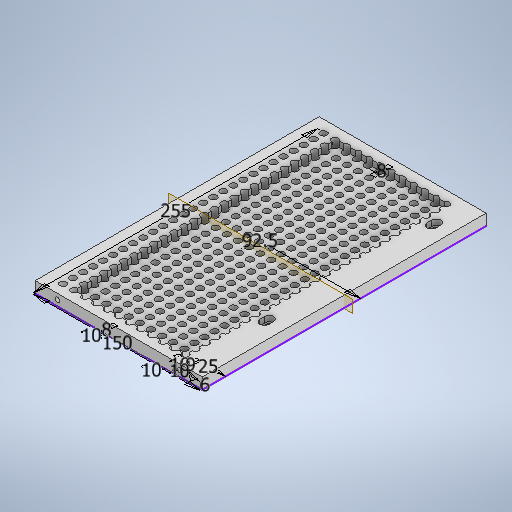
# Autodesk Inventor part: bottomplate
Saved by Autodesk Inventor 2025.2 (Build 292293000, 293)
## iProperties
Created: 2025-03-19
Part Number: bottomplate
Material: Generic
Document SubType Name: Modeling
Designer: m_kni
Density: 1 g/cm^3
Appearance: Default
Author: m_kni
Autodesk Inventor part; units mm, degrees
ref_plane "YZ Plane" through (0, 0, 0) normal (1, 0, 0) x (0, 1, 0)
ref_plane "XZ Plane" through (0, 0, 0) normal (0, 1, 0) x (-1, 0, 0)
ref_plane "XY Plane" through (0, 0, 0) normal (0, 0, 1) x (1, 0, 0)
sketch "Sketch1" plane through (0, 0, 0) normal (0, 1, 0) x (-1, 0, 0)
  line L0 (-74.8419, -127.4209) -> (75.1581, -127.4209)
  line L1 (75.1581, -127.4209) -> (75.1581, 127.5791)
  line L2 (75.1581, 127.5791) -> (-74.8419, 127.5791)
  line L3 (-74.8419, 127.5791) -> (-74.8419, -127.4209)
  line L4 (-74.8419, -127.4209) -> (75.1581, 127.5791) construction
  line L5 (75.1581, -127.4209) -> (-74.8419, 127.5791) construction
  line L6 (-74.8419, 0.0791) -> (-36.3419, 0.0791)
  line L7 (-41.3419, -127.4209) -> (-31.3419, -127.4209)
  line L8 (-31.3419, -127.4209) -> (-31.3419, 127.5791)
  line L9 (-31.3419, 127.5791) -> (-41.3419, 127.5791)
  line L10 (-41.3419, 127.5791) -> (-41.3419, -127.4209)
  line L11 (-41.3419, -127.4209) -> (-31.3419, 127.5791) construction
  line L12 (-31.3419, -127.4209) -> (-41.3419, 127.5791) construction
  line L13 (12.6581, -127.4209) -> (22.6581, -127.4209)
  line L14 (22.6581, -127.4209) -> (22.6581, 127.5791)
  line L15 (22.6581, 127.5791) -> (12.6581, 127.5791)
  line L16 (12.6581, 127.5791) -> (12.6581, -127.4209)
  line L17 (12.6581, -127.4209) -> (22.6581, 127.5791) construction
  line L18 (22.6581, -127.4209) -> (12.6581, 127.5791) construction
  line L19 (75.1581, 127.5791) -> (22.3444, 127.5791)
  line L20 (22.3444, 127.5791) -> (22.3444, 119.5791)
  line L21 (22.3444, 119.5791) -> (75.1581, 119.5791)
  line L22 (75.1581, 119.5791) -> (75.1581, 127.5791)
  line L23 (75.1581, -127.4209) -> (22.3444, -127.4209)
  line L24 (22.3444, -127.4209) -> (22.3444, -119.4209)
  line L25 (22.3444, -119.4209) -> (75.1581, -119.4209)
  line L26 (75.1581, -119.4209) -> (75.1581, -127.4209)
  line L27 (12.9719, -119.4209) -> (-31.3419, -119.4209)
  line L28 (-31.3419, -119.4209) -> (-31.3419, -127.4209)
  line L29 (-31.3419, -127.4209) -> (12.9719, -127.4209)
  line L30 (12.9719, -127.4209) -> (12.9719, -119.4209)
  line L31 (22.3444, 119.5791) -> (-31.3419, 119.5791)
  line L32 (-31.3419, 119.5791) -> (-31.3419, 127.5791)
  line L33 (-31.3419, 127.5791) -> (22.3444, 127.5791)
  line L34 (22.3444, 127.5791) -> (22.3444, 119.5791)
  point P0 (0, 0)
  point P1 (0.1581, 0.0791)
  point P2 (17.6581, 0.0791)
  point P3 (22.6581, -119.4209)
  point P4 (22.6581, 119.5791)
  point P5 (-31.3419, -119.4209)
  point P6 (12.6581, 119.5791)
  point P7 (12.6581, -119.4209)
  point P8 (-36.3419, -127.4209)
  dimension "d0" = 150
  dimension "d1" = 255
  dimension "d2" = 10
  dimension "d3" = 92.5
  dimension "d4" = 10
  dimension "d5" = 8
  dimension "d6" = 8
  constraints: 70 end point, 14 parallel, 8 horizontal, 8 midpoint, 7 perpendicular, 5 point on line
  measures "d0" distance of L2.end L1.end
  measures "d1" distance of L1.end L0.end
  measures "d2" distance of L9.end L8.end
  measures "d3" distance from line of point (17.658, 0.079) L3
  measures "d4" distance of L15.end L14.end
  measures "d5" distance of L20.end L19.end
  measures "d6" distance of L23.end L24.end
extrude "Extrusion1" add sketch "Sketch1" along normal blind 10
sketch "Sketch2" plane through (-75.1581, 0, 127.5791) normal (0, 0, 1) x (1, 0, 0)
  line L0 (0, 0) -> (0, 10) projected
  line L1 (150, 0) -> (150, 10) projected
  circle A0 centre (20, 5) radius 2.25
  circle A1 centre (130, 5) radius 2.25
  point P0 (75.1581, 0)
  point P1 (0, 5)
  point P2 (0, 5)
  point P3 (150, 5)
  dimension "d9" = 20
  dimension "d10" = 20
  dimension "d11" = 4.5
  dimension "d12" = 4.5
  constraints: 3 midpoint, 2 centre point, 2 coincident
  measures "d9" distance of point (20, 5) point (0, 5)
  measures "d10" horizontal distance of L1.start point (130, 5)
  measures "d11" diameter of A0
  measures "d12" diameter of A1
extrude "Extrusion2" cut sketch "Sketch2" against normal blind 10
ref_plane "Work Plane1" through (-75.1581, 0, 0.0791) normal (0, 0, 1) x (1, 0, 0)
mirror "Mirror1" about plane through (-75.1581, 0, 0.0791) normal (0, 0, 1) of "Extrusion2"
sketch "Sketch3" plane through (0, 0, 0) normal (0, -1, 0) x (1, 0, 0)
  line L0 (74.8419, -127.4209) -> (-75.1581, -127.4209) projected
  line L1 (74.8419, 127.5791) -> (74.8419, -127.4209) projected
  circle A0 centre (59.8419, 54.5791) radius 2.25
  circle A1 centre (59.8419, -95.4209) radius 2.25
  circle A2 centre (59.8419, -97.6709) radius 2.25
  circle A3 centre (59.8419, -93.1709) radius 2.25
  line L2 (62.0919, -93.1709) -> (62.0919, -97.6709)
  line L3 (57.5919, -93.1709) -> (57.5919, -97.6709)
  circle A4 centre (59.8419, 52.3291) radius 2.25
  circle A5 centre (59.8419, 56.8291) radius 2.25
  line L4 (57.5919, 56.8291) -> (57.5919, 52.3291)
  line L5 (62.0919, 56.8291) -> (62.0919, 52.3291)
  point P0 (0, 0)
  dimension "d15" = 32
  dimension "d16" = 15
  dimension "d17" = 150
  dimension "d19" = 4.5
  dimension "d20" = 4.5
  dimension "d21" = 4.5
  dimension "d22" = 4.5
  dimension "d23" = 4.5
  dimension "d24" = 4.5
  constraints: 12 point on circle, 8 end point, 6 centre point, 4 tangent, 1 coincident, 1 vertical
  measures "d15" distance from line of L0 point (59.842, -95.421)
  measures "d16" distance from line of L1 point (59.842, -95.421)
  measures "d17" distance of point (59.842, 54.579) point (59.842, -95.421)
  measures "d19" diameter of A0
  measures "d20" diameter of A1
  measures "d21" diameter of A2
  measures "d22" diameter of A3
  measures "d23" diameter of A4
  measures "d24" diameter of A5
extrude "Extrusion3" cut sketch "Sketch3" against normal blind 10
sketch "Sketch4" plane through (0, 10, 0) normal (0, 1, 0) x (1, 0, 0)
  line L0 (62.0919, 97.6709) -> (62.0919, 93.1709) projected
  arc A0 (57.5919, 93.1709) -> (62.0919, 93.1709) centre (59.8419, 93.1709) ccw projected
  line L1 (57.5919, 93.1709) -> (57.5919, 97.6709) projected
  arc A1 (62.0919, 97.6709) -> (57.5919, 97.6709) centre (59.8419, 97.6709) ccw projected
  line L2 (57.5919, -56.8291) -> (57.5919, -52.3291) projected
  arc A2 (62.0919, -52.3291) -> (57.5919, -52.3291) centre (59.8419, -52.3291) ccw projected
  line L3 (62.0919, -52.3291) -> (62.0919, -56.8291) projected
  arc A3 (57.5919, -56.8291) -> (62.0919, -56.8291) centre (59.8419, -56.8291) ccw projected
  line L4 (-75.1581, 127.4209) -> (-75.1581, -127.5791) projected
  line L5 (-75.1581, -127.5791) -> (74.8419, -127.5791) projected
  line L6 (74.8419, -127.5791) -> (74.8419, 127.4209) projected
  line L7 (74.8419, 127.4209) -> (-75.1581, 127.4209) projected
  circle A4 centre (59.8419, -56.8291) radius 4
  circle A5 centre (59.8419, -52.3291) radius 4
  line L8 (63.8419, -56.8291) -> (63.8419, -52.3291)
  line L9 (55.8419, -56.8291) -> (55.8419, -52.3291)
  circle A6 centre (59.8419, 93.1709) radius 4
  circle A7 centre (59.8419, 97.6709) radius 4
  line L10 (63.8419, 97.6709) -> (63.8419, 93.1709)
  line L11 (55.8419, 93.1709) -> (55.8419, 97.6709)
  point P0 (0, 0)
  point P1 (57.5919, 96.4781)
  point P2 (62.0919, 96.4781)
  dimension "d27" = 8
  dimension "d28" = 8
  dimension "d29" = 8
  dimension "d30" = 8
  constraints: 8 end point, 8 point on circle, 4 centre point, 4 coincident, 3 tangent, 2 vertical, 1 parallel
  measures "d27" diameter of A4
  measures "d28" diameter of A5
  measures "d29" diameter of A6
  measures "d30" diameter of A7
extrude "Extrusion4" cut sketch "Sketch4" against normal blind 5 contours A1 L1 A6 A7 L0 | A6 A7 L0 | L0 A7 L1 A6 | A7 A6 L1 A0 L0 | L0 A0 L1 A7 | A7 L10 A6 | L1 A7 A6 | A6 L11 A7 | A3 L3 A5 A4 L2 | A5 A4 L2 | A4 A5 L3 A2 L2 | A4 L9 A5 | L3 A4 A5 | A5 L8 A4
sketch "Sketch5" plane through (0, 10, 0) normal (0, 1, 0) x (1, 0, 0)
  line L0 (50, 117.5) -> (-50, 117.5)
  line L1 (-50, 117.5) -> (-50, -117.5)
  line L2 (-50, -117.5) -> (50, -117.5)
  line L3 (50, -117.5) -> (50, 117.5)
  line L4 (50, 117.5) -> (-50, -117.5) construction
  line L5 (-50, 117.5) -> (50, -117.5) construction
  point P0 (0, 0)
  dimension "d33" = 100
  dimension "d34" = 235
  constraints: 12 end point, 2 midpoint, 2 parallel, 1 horizontal, 1 perpendicular
  measures "d33" distance of L2.end L1.end
  measures "d34" distance of L1.end L0.end
extrude "Extrusion5" cut sketch "Sketch5" against normal up to surface (5 mm away)
sketch "Sketch6" plane through (0, 0, 0) normal (0, -1, 0) x (1, 0, 0)
  line L0 (74.8419, 127.5791) -> (74.8419, -127.4209) projected
  line L1 (-74.8419, -127.5791) -> (74.8419, -127.5791)
  line L2 (74.8419, -127.5791) -> (74.8419, 127.5791)
  line L3 (74.8419, 127.5791) -> (-74.8419, 127.5791)
  line L4 (-74.8419, 127.5791) -> (-74.8419, -127.5791)
  line L5 (-74.8419, -127.5791) -> (74.8419, 127.5791) construction
  line L6 (74.8419, -127.5791) -> (-74.8419, 127.5791) construction
  circle A0 centre (49.8419, 117.5791) radius 3
  circle A1 centre (49.8419, 108.5791) radius 3
  circle A2 centre (49.8419, 99.5791) radius 3
  circle A3 centre (49.8419, 90.5791) radius 3
  circle A4 centre (49.8419, 81.5791) radius 3
  circle A5 centre (49.8419, 72.5791) radius 3
  circle A6 centre (49.8419, 63.5791) radius 3
  circle A7 centre (49.8419, 54.5791) radius 3
  circle A8 centre (49.8419, 45.5791) radius 3
  circle A9 centre (49.8419, 36.5791) radius 3
  circle A10 centre (49.8419, 27.5791) radius 3
  circle A11 centre (49.8419, 18.5791) radius 3
  circle A12 centre (49.8419, 9.5791) radius 3
  circle A13 centre (49.8419, 0.5791) radius 3
  circle A14 centre (49.8419, -8.4209) radius 3
  circle A15 centre (49.8419, -17.4209) radius 3
  circle A16 centre (49.8419, -26.4209) radius 3
  circle A17 centre (49.8419, -35.4209) radius 3
  circle A18 centre (49.8419, -44.4209) radius 3
  circle A19 centre (49.8419, -53.4209) radius 3
  circle A20 centre (49.8419, -62.4209) radius 3
  circle A21 centre (49.8419, -71.4209) radius 3
  circle A22 centre (49.8419, -80.4209) radius 3
  circle A23 centre (49.8419, -89.4209) radius 3
  circle A24 centre (49.8419, -98.4209) radius 3
  circle A25 centre (49.8419, -107.4209) radius 3
  circle A26 centre (49.8419, -116.4209) radius 3
  circle A27 centre (39.8419, 117.5791) radius 3
  circle A28 centre (39.8419, 108.5791) radius 3
  circle A29 centre (39.8419, 99.5791) radius 3
  circle A30 centre (39.8419, 90.5791) radius 3
  circle A31 centre (39.8419, 81.5791) radius 3
  circle A32 centre (39.8419, 72.5791) radius 3
  circle A33 centre (39.8419, 63.5791) radius 3
  circle A34 centre (39.8419, 54.5791) radius 3
  circle A35 centre (39.8419, 45.5791) radius 3
  circle A36 centre (39.8419, 36.5791) radius 3
  circle A37 centre (39.8419, 27.5791) radius 3
  circle A38 centre (39.8419, 18.5791) radius 3
  circle A39 centre (39.8419, 9.5791) radius 3
  circle A40 centre (39.8419, 0.5791) radius 3
  circle A41 centre (39.8419, -8.4209) radius 3
  circle A42 centre (39.8419, -17.4209) radius 3
  circle A43 centre (39.8419, -26.4209) radius 3
  circle A44 centre (39.8419, -35.4209) radius 3
  circle A45 centre (39.8419, -44.4209) radius 3
  circle A46 centre (39.8419, -53.4209) radius 3
  circle A47 centre (39.8419, -62.4209) radius 3
  circle A48 centre (39.8419, -71.4209) radius 3
  circle A49 centre (39.8419, -80.4209) radius 3
  circle A50 centre (39.8419, -89.4209) radius 3
  circle A51 centre (39.8419, -98.4209) radius 3
  circle A52 centre (39.8419, -107.4209) radius 3
  circle A53 centre (39.8419, -116.4209) radius 3
  circle A54 centre (29.8419, 117.5791) radius 3
  circle A55 centre (29.8419, 108.5791) radius 3
  circle A56 centre (29.8419, 99.5791) radius 3
  circle A57 centre (29.8419, 90.5791) radius 3
  circle A58 centre (29.8419, 81.5791) radius 3
  circle A59 centre (29.8419, 72.5791) radius 3
  circle A60 centre (29.8419, 63.5791) radius 3
  circle A61 centre (29.8419, 54.5791) radius 3
  circle A62 centre (29.8419, 45.5791) radius 3
  circle A63 centre (29.8419, 36.5791) radius 3
  circle A64 centre (29.8419, 27.5791) radius 3
  circle A65 centre (29.8419, 18.5791) radius 3
  circle A66 centre (29.8419, 9.5791) radius 3
  circle A67 centre (29.8419, 0.5791) radius 3
  circle A68 centre (29.8419, -8.4209) radius 3
  circle A69 centre (29.8419, -17.4209) radius 3
  circle A70 centre (29.8419, -26.4209) radius 3
  circle A71 centre (29.8419, -35.4209) radius 3
  circle A72 centre (29.8419, -44.4209) radius 3
  circle A73 centre (29.8419, -53.4209) radius 3
  circle A74 centre (29.8419, -62.4209) radius 3
  circle A75 centre (29.8419, -71.4209) radius 3
  circle A76 centre (29.8419, -80.4209) radius 3
  circle A77 centre (29.8419, -89.4209) radius 3
  circle A78 centre (29.8419, -98.4209) radius 3
  circle A79 centre (29.8419, -107.4209) radius 3
  circle A80 centre (29.8419, -116.4209) radius 3
  circle A81 centre (19.8419, 117.5791) radius 3
  circle A82 centre (19.8419, 108.5791) radius 3
  circle A83 centre (19.8419, 99.5791) radius 3
  circle A84 centre (19.8419, 90.5791) radius 3
  circle A85 centre (19.8419, 81.5791) radius 3
  circle A86 centre (19.8419, 72.5791) radius 3
  circle A87 centre (19.8419, 63.5791) radius 3
  circle A88 centre (19.8419, 54.5791) radius 3
  circle A89 centre (19.8419, 45.5791) radius 3
  circle A90 centre (19.8419, 36.5791) radius 3
  circle A91 centre (19.8419, 27.5791) radius 3
  circle A92 centre (19.8419, 18.5791) radius 3
  circle A93 centre (19.8419, 9.5791) radius 3
  circle A94 centre (19.8419, 0.5791) radius 3
  circle A95 centre (19.8419, -8.4209) radius 3
  circle A96 centre (19.8419, -17.4209) radius 3
  circle A97 centre (19.8419, -26.4209) radius 3
  circle A98 centre (19.8419, -35.4209) radius 3
  circle A99 centre (19.8419, -44.4209) radius 3
  circle A100 centre (19.8419, -53.4209) radius 3
  circle A101 centre (19.8419, -62.4209) radius 3
  circle A102 centre (19.8419, -71.4209) radius 3
  circle A103 centre (19.8419, -80.4209) radius 3
  circle A104 centre (19.8419, -89.4209) radius 3
  circle A105 centre (19.8419, -98.4209) radius 3
  circle A106 centre (19.8419, -107.4209) radius 3
  circle A107 centre (19.8419, -116.4209) radius 3
  circle A108 centre (9.8419, 117.5791) radius 3
  circle A109 centre (9.8419, 108.5791) radius 3
  circle A110 centre (9.8419, 99.5791) radius 3
  circle A111 centre (9.8419, 90.5791) radius 3
  circle A112 centre (9.8419, 81.5791) radius 3
  circle A113 centre (9.8419, 72.5791) radius 3
  circle A114 centre (9.8419, 63.5791) radius 3
  circle A115 centre (9.8419, 54.5791) radius 3
  circle A116 centre (9.8419, 45.5791) radius 3
  circle A117 centre (9.8419, 36.5791) radius 3
  circle A118 centre (9.8419, 27.5791) radius 3
  circle A119 centre (9.8419, 18.5791) radius 3
  circle A120 centre (9.8419, 9.5791) radius 3
  circle A121 centre (9.8419, 0.5791) radius 3
  circle A122 centre (9.8419, -8.4209) radius 3
  circle A123 centre (9.8419, -17.4209) radius 3
  circle A124 centre (9.8419, -26.4209) radius 3
  circle A125 centre (9.8419, -35.4209) radius 3
  circle A126 centre (9.8419, -44.4209) radius 3
  circle A127 centre (9.8419, -53.4209) radius 3
  circle A128 centre (9.8419, -62.4209) radius 3
  circle A129 centre (9.8419, -71.4209) radius 3
  circle A130 centre (9.8419, -80.4209) radius 3
  circle A131 centre (9.8419, -89.4209) radius 3
  circle A132 centre (9.8419, -98.4209) radius 3
  circle A133 centre (9.8419, -107.4209) radius 3
  circle A134 centre (9.8419, -116.4209) radius 3
  circle A135 centre (-0.1581, 117.5791) radius 3
  circle A136 centre (-0.1581, 108.5791) radius 3
  circle A137 centre (-0.1581, 99.5791) radius 3
  circle A138 centre (-0.1581, 90.5791) radius 3
  circle A139 centre (-0.1581, 81.5791) radius 3
  circle A140 centre (-0.1581, 72.5791) radius 3
  circle A141 centre (-0.1581, 63.5791) radius 3
  circle A142 centre (-0.1581, 54.5791) radius 3
  circle A143 centre (-0.1581, 45.5791) radius 3
  circle A144 centre (-0.1581, 36.5791) radius 3
  circle A145 centre (-0.1581, 27.5791) radius 3
  circle A146 centre (-0.1581, 18.5791) radius 3
  circle A147 centre (-0.1581, 9.5791) radius 3
  circle A148 centre (-0.1581, 0.5791) radius 3
  circle A149 centre (-0.1581, -8.4209) radius 3
  circle A150 centre (-0.1581, -17.4209) radius 3
  circle A151 centre (-0.1581, -26.4209) radius 3
  circle A152 centre (-0.1581, -35.4209) radius 3
  circle A153 centre (-0.1581, -44.4209) radius 3
  circle A154 centre (-0.1581, -53.4209) radius 3
  circle A155 centre (-0.1581, -62.4209) radius 3
  circle A156 centre (-0.1581, -71.4209) radius 3
  circle A157 centre (-0.1581, -80.4209) radius 3
  circle A158 centre (-0.1581, -89.4209) radius 3
  circle A159 centre (-0.1581, -98.4209) radius 3
  circle A160 centre (-0.1581, -107.4209) radius 3
  circle A161 centre (-0.1581, -116.4209) radius 3
  circle A162 centre (-10.1581, 117.5791) radius 3
  circle A163 centre (-10.1581, 108.5791) radius 3
  circle A164 centre (-10.1581, 99.5791) radius 3
  circle A165 centre (-10.1581, 90.5791) radius 3
  circle A166 centre (-10.1581, 81.5791) radius 3
  circle A167 centre (-10.1581, 72.5791) radius 3
  circle A168 centre (-10.1581, 63.5791) radius 3
  circle A169 centre (-10.1581, 54.5791) radius 3
  circle A170 centre (-10.1581, 45.5791) radius 3
  circle A171 centre (-10.1581, 36.5791) radius 3
  circle A172 centre (-10.1581, 27.5791) radius 3
  circle A173 centre (-10.1581, 18.5791) radius 3
  circle A174 centre (-10.1581, 9.5791) radius 3
  circle A175 centre (-10.1581, 0.5791) radius 3
  circle A176 centre (-10.1581, -8.4209) radius 3
  circle A177 centre (-10.1581, -17.4209) radius 3
  circle A178 centre (-10.1581, -26.4209) radius 3
  circle A179 centre (-10.1581, -35.4209) radius 3
  circle A180 centre (-10.1581, -44.4209) radius 3
  circle A181 centre (-10.1581, -53.4209) radius 3
  circle A182 centre (-10.1581, -62.4209) radius 3
  circle A183 centre (-10.1581, -71.4209) radius 3
  circle A184 centre (-10.1581, -80.4209) radius 3
  circle A185 centre (-10.1581, -89.4209) radius 3
  circle A186 centre (-10.1581, -98.4209) radius 3
  circle A187 centre (-10.1581, -107.4209) radius 3
  circle A188 centre (-10.1581, -116.4209) radius 3
  circle A189 centre (-20.1581, 117.5791) radius 3
  circle A190 centre (-20.1581, 108.5791) radius 3
  circle A191 centre (-20.1581, 99.5791) radius 3
  circle A192 centre (-20.1581, 90.5791) radius 3
  circle A193 centre (-20.1581, 81.5791) radius 3
  circle A194 centre (-20.1581, 72.5791) radius 3
  circle A195 centre (-20.1581, 63.5791) radius 3
  circle A196 centre (-20.1581, 54.5791) radius 3
  circle A197 centre (-20.1581, 45.5791) radius 3
  circle A198 centre (-20.1581, 36.5791) radius 3
  circle A199 centre (-20.1581, 27.5791) radius 3
  circle A200 centre (-20.1581, 18.5791) radius 3
  circle A201 centre (-20.1581, 9.5791) radius 3
  circle A202 centre (-20.1581, 0.5791) radius 3
  circle A203 centre (-20.1581, -8.4209) radius 3
  circle A204 centre (-20.1581, -17.4209) radius 3
  circle A205 centre (-20.1581, -26.4209) radius 3
  circle A206 centre (-20.1581, -35.4209) radius 3
  circle A207 centre (-20.1581, -44.4209) radius 3
  circle A208 centre (-20.1581, -53.4209) radius 3
  circle A209 centre (-20.1581, -62.4209) radius 3
  circle A210 centre (-20.1581, -71.4209) radius 3
  circle A211 centre (-20.1581, -80.4209) radius 3
  circle A212 centre (-20.1581, -89.4209) radius 3
  circle A213 centre (-20.1581, -98.4209) radius 3
  circle A214 centre (-20.1581, -107.4209) radius 3
  circle A215 centre (-20.1581, -116.4209) radius 3
  circle A216 centre (-30.1581, 117.5791) radius 3
  circle A217 centre (-30.1581, 108.5791) radius 3
  circle A218 centre (-30.1581, 99.5791) radius 3
  circle A219 centre (-30.1581, 90.5791) radius 3
  circle A220 centre (-30.1581, 81.5791) radius 3
  circle A221 centre (-30.1581, 72.5791) radius 3
  circle A222 centre (-30.1581, 63.5791) radius 3
  circle A223 centre (-30.1581, 54.5791) radius 3
  circle A224 centre (-30.1581, 45.5791) radius 3
  circle A225 centre (-30.1581, 36.5791) radius 3
  circle A226 centre (-30.1581, 27.5791) radius 3
  circle A227 centre (-30.1581, 18.5791) radius 3
  circle A228 centre (-30.1581, 9.5791) radius 3
  circle A229 centre (-30.1581, 0.5791) radius 3
  circle A230 centre (-30.1581, -8.4209) radius 3
  circle A231 centre (-30.1581, -17.4209) radius 3
  circle A232 centre (-30.1581, -26.4209) radius 3
  circle A233 centre (-30.1581, -35.4209) radius 3
  circle A234 centre (-30.1581, -44.4209) radius 3
  circle A235 centre (-30.1581, -53.4209) radius 3
  circle A236 centre (-30.1581, -62.4209) radius 3
  circle A237 centre (-30.1581, -71.4209) radius 3
  circle A238 centre (-30.1581, -80.4209) radius 3
  circle A239 centre (-30.1581, -89.4209) radius 3
  circle A240 centre (-30.1581, -98.4209) radius 3
  circle A241 centre (-30.1581, -107.4209) radius 3
  circle A242 centre (-30.1581, -116.4209) radius 3
  circle A243 centre (-40.1581, 117.5791) radius 3
  circle A244 centre (-40.1581, 108.5791) radius 3
  circle A245 centre (-40.1581, 99.5791) radius 3
  circle A246 centre (-40.1581, 90.5791) radius 3
  circle A247 centre (-40.1581, 81.5791) radius 3
  circle A248 centre (-40.1581, 72.5791) radius 3
  circle A249 centre (-40.1581, 63.5791) radius 3
  circle A250 centre (-40.1581, 54.5791) radius 3
  circle A251 centre (-40.1581, 45.5791) radius 3
  circle A252 centre (-40.1581, 36.5791) radius 3
  circle A253 centre (-40.1581, 27.5791) radius 3
  circle A254 centre (-40.1581, 18.5791) radius 3
  circle A255 centre (-40.1581, 9.5791) radius 3
  circle A256 centre (-40.1581, 0.5791) radius 3
  circle A257 centre (-40.1581, -8.4209) radius 3
  circle A258 centre (-40.1581, -17.4209) radius 3
  circle A259 centre (-40.1581, -26.4209) radius 3
  circle A260 centre (-40.1581, -35.4209) radius 3
  circle A261 centre (-40.1581, -44.4209) radius 3
  circle A262 centre (-40.1581, -53.4209) radius 3
  circle A263 centre (-40.1581, -62.4209) radius 3
  circle A264 centre (-40.1581, -71.4209) radius 3
  circle A265 centre (-40.1581, -80.4209) radius 3
  circle A266 centre (-40.1581, -89.4209) radius 3
  circle A267 centre (-40.1581, -98.4209) radius 3
  circle A268 centre (-40.1581, -107.4209) radius 3
  circle A269 centre (-40.1581, -116.4209) radius 3
  circle A270 centre (-50.1581, 117.5791) radius 3
  circle A271 centre (-50.1581, 108.5791) radius 3
  circle A272 centre (-50.1581, 99.5791) radius 3
  circle A273 centre (-50.1581, 90.5791) radius 3
  circle A274 centre (-50.1581, 81.5791) radius 3
  circle A275 centre (-50.1581, 72.5791) radius 3
  circle A276 centre (-50.1581, 63.5791) radius 3
  circle A277 centre (-50.1581, 54.5791) radius 3
  circle A278 centre (-50.1581, 45.5791) radius 3
  circle A279 centre (-50.1581, 36.5791) radius 3
  circle A280 centre (-50.1581, 27.5791) radius 3
  circle A281 centre (-50.1581, 18.5791) radius 3
  circle A282 centre (-50.1581, 9.5791) radius 3
  circle A283 centre (-50.1581, 0.5791) radius 3
  circle A284 centre (-50.1581, -8.4209) radius 3
  circle A285 centre (-50.1581, -17.4209) radius 3
  circle A286 centre (-50.1581, -26.4209) radius 3
  circle A287 centre (-50.1581, -35.4209) radius 3
  circle A288 centre (-50.1581, -44.4209) radius 3
  circle A289 centre (-50.1581, -53.4209) radius 3
  circle A290 centre (-50.1581, -62.4209) radius 3
  circle A291 centre (-50.1581, -71.4209) radius 3
  circle A292 centre (-50.1581, -80.4209) radius 3
  circle A293 centre (-50.1581, -89.4209) radius 3
  circle A294 centre (-50.1581, -98.4209) radius 3
  circle A295 centre (-50.1581, -107.4209) radius 3
  circle A296 centre (-50.1581, -116.4209) radius 3
  circle A297 centre (-60.1581, 117.5791) radius 3
  circle A298 centre (-60.1581, 108.5791) radius 3
  circle A299 centre (-60.1581, 99.5791) radius 3
  circle A300 centre (-60.1581, 90.5791) radius 3
  circle A301 centre (-60.1581, 81.5791) radius 3
  circle A302 centre (-60.1581, 72.5791) radius 3
  circle A303 centre (-60.1581, 63.5791) radius 3
  circle A304 centre (-60.1581, 54.5791) radius 3
  circle A305 centre (-60.1581, 45.5791) radius 3
  circle A306 centre (-60.1581, 36.5791) radius 3
  circle A307 centre (-60.1581, 27.5791) radius 3
  circle A308 centre (-60.1581, 18.5791) radius 3
  circle A309 centre (-60.1581, 9.5791) radius 3
  circle A310 centre (-60.1581, 0.5791) radius 3
  circle A311 centre (-60.1581, -8.4209) radius 3
  circle A312 centre (-60.1581, -17.4209) radius 3
  circle A313 centre (-60.1581, -26.4209) radius 3
  circle A314 centre (-60.1581, -35.4209) radius 3
  circle A315 centre (-60.1581, -44.4209) radius 3
  circle A316 centre (-60.1581, -53.4209) radius 3
  circle A317 centre (-60.1581, -62.4209) radius 3
  circle A318 centre (-60.1581, -71.4209) radius 3
  circle A319 centre (-60.1581, -80.4209) radius 3
  circle A320 centre (-60.1581, -89.4209) radius 3
  circle A321 centre (-60.1581, -98.4209) radius 3
  circle A322 centre (-60.1581, -107.4209) radius 3
  circle A323 centre (-60.1581, -116.4209) radius 3
  point P0 (0, 0)
  dimension "d37" = 6
  dimension "d38" = 10
  dimension "d39" = 25
  dimension "d42" = 9
  dimension "d45" = 10
  constraints: 324 centre point, 12 end point, 2 horizontal, 2 midpoint, 2 parallel, 1 perpendicular, 1 vertical, 646 other
  measures "d37" diameter of A0
  measures "d38" distance from line of A0.centre L3
  measures "d39" distance from line of L0 A0.centre
  measures "d42" distance of A0.centre A1.centre
  measures "d45" distance of A0.centre A27.centre
extrude "Extrusion7" cut sketch "Sketch6" against normal blind 10 contours A0 | A1 | A2 | A3 | A4 | A5 | A6 | A7 | A8 | A9 | A10 | A11 | A12 | A27 | A28 | A29 | A30 | A31 | A32 | A33 | A34 | A35 | A36 | A37 | A38 | A39 | A54 | A55 | A56 | A57 | A58 | A59 | A60 | A61 | A62 | A63 | A64 | A65 | A66 | A81 | A82 | A83 | A84 | A85 | A86 | A87 | A88 | A89 | A90 | A91 | A92 | A93 | A108 | A109 | A110 | A111 | A112 | A113 | A114 | A115 | A116 | A117 | A118 | A119 | A120 | A135 | A136 | A137 | A138 | A139 | A140 | A141 | A142 | A143 | A144 | A145 | A146 | A147 | A162 | A163 | A164 | A165 | A166 | A167 | A168 | A169 | A170 | A171 | A172 | A173 | A174 | A189 | A190 | A191 | A192 | A193 | A194 | A195 | A196 | A197 | A198 | A199 | A200 | A201 | A216 | A217 | A218 | A219 | A220 | A221 | A222 | A223 | A224 | A225 | A226 | A227 | A228 | A243 | A244 | A245 | A246 | A247 | A248 | A249 | A250 | A251 | A252 | A253 | A254 | A255 | A270 | A271 | A272 | A273 | A274 | A275 | A276 | A277 | A278 | A279 | A280 | A281 | A282 | A283 | A284 | A285 | A286 | A287 | A288 | A289 | A290 | A291 | A292 | A293 | A294 | A295 | A296 | A297 | A298 | A299 | A300 | A301 | A302 | A303 | A304 | A305 | A306 | A307 | A308 | A309 | A310 | A311 | A312 | A313 | A314 | A315 | A316 | A317 | A318 | A319 | A320 | A321 | A322 | A323
extrude "Extrusion8" cut sketch "Sketch6" against normal blind 92.5 contours A13 | A14 | A15 | A16 | A17 | A18 | A19 | A20 | A21 | A22 | A23 | A24 | A25 | A26 | A40 | A41 | A42 | A43 | A44 | A45 | A46 | A47 | A48 | A49 | A50 | A51 | A52 | A53 | A67 | A68 | A69 | A70 | A71 | A72 | A73 | A74 | A75 | A76 | A77 | A78 | A79 | A80 | A94 | A95 | A96 | A97 | A98 | A99 | A100 | A101 | A102 | A103 | A104 | A105 | A106 | A107 | A121 | A122 | A123 | A124 | A125 | A126 | A127 | A128 | A129 | A130 | A131 | A132 | A133 | A134 | A148 | A149 | A150 | A151 | A152 | A153 | A154 | A155 | A156 | A157 | A158 | A159 | A160 | A161 | A175 | A176 | A177 | A178 | A179 | A180 | A181 | A182 | A183 | A184 | A185 | A186 | A187 | A188 | A202 | A203 | A204 | A205 | A206 | A207 | A208 | A209 | A210 | A211 | A212 | A213 | A214 | A215 | A229 | A230 | A231 | A232 | A233 | A234 | A235 | A236 | A237 | A238 | A239 | A240 | A241 | A242 | A256 | A257 | A258 | A259 | A260 | A261 | A262 | A263 | A264 | A265 | A266 | A267 | A268 | A269
body "Solid1"
